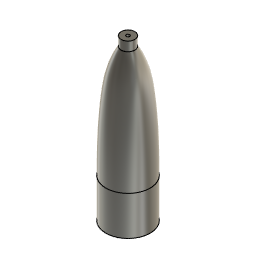
KAISO_6 (Autodesk Fusion 360 design; units mm, degrees)
Autodesk Fusion 360 part; units mm, degrees
sketch "スケッチ1" plane through (0, 0, 0) normal (0, 1, 0) x (1, 0, 0)
  line L0 (0, -55) -> (-1.4, -55)
  line L1 (0, -55) -> (0, -155.1583)
  line L2 (0, -178.5668) -> (0, 150)
  spline S0 degree 5 poles (-1.4, -55) (-1.7809, -54.235) (-2.4752, -52.7476) (-3.3143, -50.6447) (-4.0727, -48.0276) (-4.6457, -44.727) (-5.066, -41.1251) (-5.4831, -37.1291) (-5.7992, -33.2634) (-5.99, -29.5181) (-6.0766, -25.5762) (-6.0952, -21.9015) (-6.0991, -18.6627) (-6.1, -16.2613) (-6.1, -15) knots 0 0 0 0 0 0 0.1 0.2 0.3 0.4 0.5 0.6 0.7 0.8 0.9 1 1 1 1 1 1
  line L3 (0.7611, -59.3408) -> (-3.5611, -50.6592)
  line L4 (-6.1, -21) -> (-6.1, -9)
  line L5 (0, -60) -> (-0.8, -60)
  spline S1 degree 5 poles (-8.5, -15) (-8.5, -15.6448) (-8.4987, -16.9599) (-8.4927, -19.0086) (-8.473, -21.8929) (-8.4091, -25.7404) (-8.2819, -29.791) (-8.0713, -33.9618) (-7.7678, -38.1111) (-7.3809, -42.015) (-6.9485, -45.348) (-6.4546, -48.139) (-5.8649, -50.5502) (-5.1393, -52.7932) (-4.2509, -55.009) (-3.2096, -57.1277) (-2.2833, -58.5651) (-1.5531, -59.3938) (-1.0532, -59.8191) (-0.8, -60) knots 0 0 0 0 0 0 0.066667 0.133333 0.2 0.266667 0.333333 0.4 0.466667 0.533333 0.6 0.666667 0.733333 0.8 0.866667 0.933333 1 1 1 1 1 1
  line L6 (-8.1174, -34.3114) -> (-7.0765, -45.085)
  line L7 (-8.5, -11) -> (-8.5, -19)
  line L8 (-3.6, -58) -> (2, -62)
  line L9 (-4.8933, -42.8286) -> (-5.7034, -34.7953)
  line L10 (-2.6346, -59.5) -> (-2.6346, -60.5)
  line L11 (-2.6346, -59.5) -> (-2.6346, -57.9467)
  line L12 (-2.6346, -60.5) -> (-2.6346, -61.5)
  line L13 (-2.6346, -61.5) -> (0, -61.5)
  line L14 (-8.5, -15) -> (-8.5, 0)
  line L15 (-8.5, 0) -> (-6.1, 0)
  line L16 (-6.1, 0) -> (-6.1, -15)
  point P0 (-6.1, 0)
  point P1 (0, -60)
  point P2 (230, -390)
  point P3 (0, -55)
  point P4 (-1.4, -55)
  point P5 (-5.2983, -38.8119)
  point P6 (-7.597, -39.6982)
  point P7 (-4.8404, -53.4752)
  dimension "d1" = 6.1
  dimension "d3" = 60
  dimension "d6" = 5
  dimension "d7" = 1.4
  dimension "d14" = 0.8
  constraint coincident P3 L0.start
  constraint coincident P4 L0.end
  constraint perpendicular L0 L1
  constraint perpendicular L0 L2
  constraint midpoint P4 L3
  constraint midpoint S0.end L4
  constraint coincident P1 L5.start
  constraint perpendicular L2 L5
  constraint midpoint P6 L6
  constraint midpoint S1.start L7
  constraint midpoint L5.end L8
  constraint midpoint P5 L9
  constraint perpendicular L5 L10
  constraint coincident S1 L11.end
  constraint perpendicular L5 L11
  constraint parallel L10 L12
  constraint coincident L1 L13.end
  constraint coincident L2 L13.end
  constraint vertical L14
  constraint coincident P0 L15.end
  constraint perpendicular L14 L15
  constraint perpendicular L15 L16
  measures "d1" distance of origin P0
  measures "d3" distance of origin L5.start
  measures "d6" distance of P1 L0.start
  measures "d7" distance of P3 P4
  measures "d14" distance of P1 L5.end
revolve "回転1" add sketch "スケッチ1" angle 360 about axis through (0, 0, 178.5668) along (0, 0, -1)
sketch "スケッチ3" plane through (0, 0, 55) normal (0, 0, -1) x (1, 0, 0)
  circle A0 centre (0, 0) radius 1.4
  constraint coincident A0.centre origin
hole "穴1" at (0, 0, 55) direction (0, 0, 1) diameter 1.3 depth 250 tip angle 118
revolve "回転2" add sketch "スケッチ1" angle 360 about axis through (0, 0, 178.5668) along (0, 0, -1) contours L0 L1 L2 L3 | L1 L2 S0 L3 L4 L5 S1 L7 L14 L15 L16
